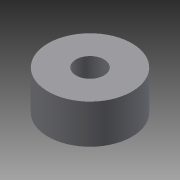
# Autodesk Inventor part: 10mm-single
Saved by Autodesk Inventor 2013 (Build 170138000, 138)
## iProperties
Created: 2012-12-06
Part Number: 10mm-single
Material: Generic
Document SubType Name: Modeling
Designer: Istvan
Density: 1 g/cm^3
Mass: 1.8099 g
Surface Area: 10.7675 cm^2
Volume: 1.8099 cm^3
Author: Istvan
Autodesk Inventor part; units mm, degrees
ref_plane "YZ Plane" through (0, 0, 0) normal (1, 0, 0) x (0, 1, 0)
ref_plane "XZ Plane" through (0, 0, 0) normal (0, 1, 0) x (-1, 0, 0)
ref_plane "XY Plane" through (0, 0, 0) normal (0, 0, 1) x (1, 0, 0)
sketch "Sketch1" plane through (0, 0, 0) normal (0, 1, 0) x (-1, 0, 0)
  circle A0 centre (0, 0) radius 5
  circle A1 centre (0, 0) radius 15
  dimension "d0" = 10
  dimension "d1" = 30
  constraints: 2 centre point, 2 coincident
  measures "d0" diameter of A0
  measures "d1" diameter of A1
extrude "Extrusion1" add sketch "Sketch1" along normal blind 14
body "Solid1"
